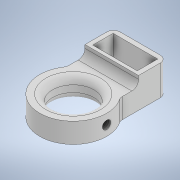
# Autodesk Inventor part: Final Carrera Y0
Saved by Autodesk Inventor 2021 (Build 250183000, 183)
## iProperties
Created: 2022-09-17
Part Number: Final Carrera Y0
Material: Genérico
Document SubType Name: Modeling
Designer: sergi
Density: 1 g/cm^3
Appearance: Valor por defecto
Author: sergi
Autodesk Inventor part; units mm, degrees
ref_plane "YZ Plane" through (0, 0, 0) normal (1, 0, 0) x (0, 1, 0)
sketch "Boceto1" plane through (0, 0, 0) normal (0, 1, 0) x (-1, 0, 0)
  circle A0 centre (0, 0) radius 10
  dimension "d0" = 20
  constraints: 1 centre point, 1 coincident
  measures "d0" diameter of A0
extrude "Extrusión1" add sketch "Boceto1" along normal blind 6
ref_plane "Plano de trabajo6" through (0, 0, -10) normal (0, 0, 1) x (1, 0, 0)
sketch "Boceto3" plane through (0, 0, -10) normal (0, 0, 1) x (1, 0, 0)
  line L0 (10, 0) -> (-10, 0) projected
  line L1 (8, 0) -> (8, 10)
  line L2 (10, 10) -> (-10, 10) projected
  line L3 (8, 10) -> (-8, 10)
  line L4 (-8, 10) -> (-8, 0)
  line L5 (-8, 0) -> (8, 0)
  point P0 (0, 0)
  dimension "d10" = 8
  dimension "d11" = 10
  dimension "d12" = 16
  constraints: 8 end point, 3 point on line, 2 collinear, 1 perpendicular
  measures "d10" distance of point (0, 0) L1.start
  measures "d11" distance of L1.start L1.end
  measures "d12" distance of L1.end L3.end
extrude "Extrusión2" add sketch "Boceto3" along normal blind 5 and the other way blind 7
sketch "Boceto4" plane through (0, 6, 0) normal (0, 1, 0) x (1, 0, 0)
  line L0 (-8, 17) -> (8, 17) projected
  line L1 (-6.7, 15.6) -> (6.6, 15.6)
  line L2 (6.6, 15.6) -> (6.6, 9.5)
  line L3 (6.6, 9.5) -> (-6.7, 9.5)
  line L4 (-6.7, 9.5) -> (-6.7, 15.6)
  line L5 (-6.6, 18.5) -> (6.6, 12.5) construction
  line L6 (6.6, 18.5) -> (-6.6, 12.5) construction
  point P0 (0, 0)
  dimension "d19" = 13.3
  dimension "d20" = 6.1
  constraints: 12 end point, 2 parallel, 1 horizontal, 1 perpendicular
  measures "d19" distance of L2.end L3.end
  measures "d20" distance of L1.end L2.end
extrude "Extrusión3" cut sketch "Boceto4" against normal blind 10
sketch "Boceto5" plane through (0, 6, 0) normal (0, 1, 0) x (1, 0, 0)
  arc A0 (-8, 6) -> (8, 6) centre (0, 0) ccw projected
  constraints: 1 coincident
hole "Agujero2" at (0, 6, 0) direction (0, -1, 0) diameter 12.3 end through all
ref_plane "Plano de trabajo5" through (10, 0, 0) normal (1, 0, 0) x (0, 1, 0)
sketch "Boceto6" plane through (10, 0, 0) normal (1, 0, 0) x (0, 1, 0)
  line L0 (0, 0) -> (3, 0)
  dimension "d32" = 3
  constraints: 2 end point, 1 horizontal
  measures "d32" distance of L0.start L0.end
hole "Agujero3" at (10, 3, 0) direction (-1, 0, 0) diameter 2.459 depth 5 thread size "M3x0.5" class "6H" standard "ANSI Metric M Profile"
sketch "Boceto7" plane through (0, 0, -5) normal (0, 0, 1) x (1, 0, 0)
  line L0 (-8, 6) -> (-8.3333, 6) projected
  line L1 (8, 10) -> (-8, 10)
  line L2 (-8, 10) -> (-8, 6)
  line L3 (-8, 6) -> (8, 6)
  line L4 (8, 6) -> (8, 10)
  point P0 (0, 0)
  constraints: 8 end point, 2 parallel, 1 horizontal, 1 perpendicular
extrude "Extrusión4" cut sketch "Boceto7" against normal blind 17
fillet "Empalme4" radius 2 2 edges at (0, 6, -6.15) (0, 0, -6.15)
sketch "Boceto8" plane through (0, 6, 0) normal (0, 1, 0) x (1, 0, 0)
  line L0 (-8, 6) -> (-8, 17) projected
  line L1 (-8, 17) -> (8, 17)
  line L2 (8, 17) -> (8, 8.5)
  line L3 (8, 8.5) -> (-8, 8.5)
  line L4 (-8, 8.5) -> (-8, 17)
  point P0 (0, 0)
  dimension "d45" = 16
  dimension "d46" = 8.5
  constraints: 8 end point, 2 parallel, 1 horizontal, 1 perpendicular
  measures "d45" distance of L2.end L3.end
  measures "d46" distance of L1.end L2.end
extrude "Extrusión5" add sketch "Boceto8" along normal blind 3
sketch "Boceto9" plane through (0, 0, -17) normal (0, 0, -1) x (-1, 0, 0)
  line L0 (-8, 9) -> (-8, 0) projected
  line L1 (8, 0) -> (8, 9) projected
  line L2 (-8, 9) -> (8, 9)
  line L3 (8, 9) -> (8, 0)
  line L4 (8, 0) -> (-8, 0)
  line L5 (-8, 0) -> (-8, 9)
  point P0 (0, 0)
  constraints: 8 end point, 2 parallel, 1 horizontal, 1 perpendicular
extrude "Extrusión6" add sketch "Boceto9" along normal blind 3
sketch "Boceto10" plane through (6.6, 0, -9.5) normal (0, 0, -1) x (-1, 0, 0)
  line L0 (0, 6) -> (0, 0) projected
  line L1 (13.3, 6) -> (13.3, 0) projected
  line L2 (0, 6) -> (13.3, 6)
  line L3 (13.3, 6) -> (13.3, 0)
  line L4 (13.3, 0) -> (0, 0)
  line L5 (0, 0) -> (0, 6)
  point P0 (6.6, 0)
  constraints: 8 end point, 2 parallel, 1 horizontal, 1 perpendicular
extrude "Extrusión7" add sketch "Boceto10" along normal blind 3
sketch "Boceto11" plane through (-6.7, 0, -15.6) normal (0, 0, 1) x (1, 0, 0)
  line L0 (13.3, 6) -> (0, 6) projected
  line L1 (13.3, 0) -> (0, 0) projected
  line L2 (0, 6) -> (13.3, 6)
  line L3 (13.3, 6) -> (13.3, 0)
  line L4 (13.3, 0) -> (0, 0)
  line L5 (0, 0) -> (0, 6)
  point P0 (6.7, 0)
  constraints: 8 end point, 2 parallel, 1 horizontal, 1 perpendicular
extrude "Extrusión8" cut sketch "Boceto11" against normal blind 3
sketch "Boceto12" plane through (-8, 6, -8.5) normal (0, 0, 1) x (1, 0, 0)
  line L0 (16, 0) -> (16, 3) projected
  line L1 (16, 3) -> (0, 3)
  line L2 (0, 3) -> (0, 0)
  line L3 (0, 0) -> (16, 0)
  line L4 (16, 0) -> (16, 3)
  point P0 (8, -6)
  constraints: 8 end point, 2 parallel, 1 horizontal, 1 perpendicular
extrude "Extrusión9" cut sketch "Boceto12" against normal blind 3
sketch "Boceto13" plane through (0, 6, 0) normal (0, -1, 0) x (1, 0, 0)
  line L0 (6.6, -12.5) -> (-6.7, -12.5) projected
  line L1 (-6.7, -12.5) -> (-6.7, -18.6) projected
  line L2 (6.6, -12.5) -> (-6.7, -12.5)
  line L3 (-6.7, -12.5) -> (-6.7, -18.6)
  line L4 (-6.7, -18.6) -> (6.6, -18.6)
  line L5 (6.6, -18.6) -> (6.6, -12.5)
  point P0 (0, 0)
  constraints: 8 end point, 2 parallel, 1 horizontal, 1 perpendicular
extrude "Extrusión10" cut sketch "Boceto13" against normal blind 3
fillet "Empalme5" radius 2 4 edges at (8, 4.5, -20) (-8, 4.5, -20) (-8, 3, -6) (8, 3, -6)
fillet "Empalme6" radius 2 1 edges at (0, 6, -11.5)
